37mm Analog Hygrometer or Thermometer (Autodesk Fusion 360 design; units mm, degrees)
Autodesk Fusion 360 part; units mm, degrees
sketch "Sketch1" plane through (0, 0, 0) normal (0, 1, 0) x (1, 0, 0)
  line L0 (8.4, 0) -> (15.75, 0)
  line L1 (15.75, 0) -> (15.85, -7.5)
  line L2 (15.85, -7.5) -> (18.5, -7.5)
  line L3 (18.5, -7.5) -> (18.5, -8.8)
  line L4 (18.5, -8.8) -> (15, -9.8)
  line L5 (15, -9.8) -> (0, -9.8)
  line L6 (0, -9.8) -> (0, -0.35)
  line L7 (8.4, 0) -> (8.4, -0.35)
  line L8 (8.4, -0.35) -> (0, -0.35)
  dimension "d2" = 15.85
  dimension "d3" = 15.75
  dimension "d4" = 7.5
  dimension "d5" = 18.5
  dimension "d6" = 9.8
  dimension "d7" = 15
  dimension "d8" = 1.3
  dimension "d9" = 0.35
  dimension "d10" = 8.4
  constraint horizontal L0
  constraint parallel L0 L2
  constraint perpendicular L2 L3
  constraint parallel L2 L5
  constraint perpendicular L0 L6
  constraint perpendicular L0 L7
  constraint perpendicular L6 L8
  constraint coincident origin L0
  constraint coincident origin L6
  measures "d2" distance of L1.end L6
  measures "d3" distance of origin L0.end
  measures "d4" distance of L0.end L2
  measures "d5" distance of L3 L6
  measures "d6" distance of origin L5.end
  measures "d7" distance of L4.end L5.end
  measures "d8" distance of L2.end L3.end
  measures "d9" distance of L0.start L7.end
  measures "d10" distance of L7.end L6.end
revolve "Revolve1" add sketch "Sketch1" angle 360 about axis through (0, 0, 9.8) along (0, 0, -1)
equation "d2 = ( 31.7 / 2 ) * 1 mm"
equation "d3 = ( 31.5 / 2 ) * 1 mm"
equation "d5 = ( 37 / 2 ) * 1 mm"
equation "d10 = ( 16.8 / 2 ) * 1 mm"
